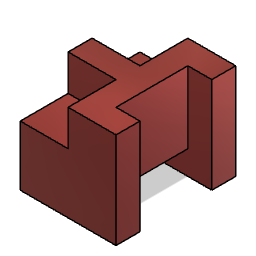
3d09 v1 (Autodesk Fusion 360 design; units mm, degrees)
Autodesk Fusion 360 part; units mm, degrees
sketch "Sketch1" plane through (0, 0, 0) normal (0, 0, 1) x (1, 0, 0)
  line L0 (0, 0) -> (0, 25)
  line L1 (0, 25) -> (20, 25)
  line L2 (20, 25) -> (20, 40)
  line L3 (20, 40) -> (40, 40)
  line L4 (40, 40) -> (40, 0)
  line L5 (40, 0) -> (0, 0)
  dimension "d1" = 40
  dimension "d2" = 25
  dimension "d3" = 20
  dimension "d4" = 15
  constraint coincident L0.start L5.end
  constraint vertical L0
  constraint perpendicular L0 L1
  constraint perpendicular L1 L2
  constraint perpendicular L2 L3
  constraint perpendicular L3 L4
  constraint perpendicular L0 L5
  measures "d1" distance of L4.end L0.start
  measures "d2" distance of L0.start L0.end
  measures "d3" distance of L2.end L3.end
  measures "d4" distance of L1.end L2.end
extrude "Extrude1" add sketch "Sketch1" along normal mid plane 50
sketch "Sketch2" plane through (0, 0, 0) normal (0, 0, 1) x (1, 0, 0)
  line L0 (0, 40) -> (20, 40)
  line L1 (20, 40) -> (20, 25)
  line L2 (20, 25) -> (0, 25)
  line L3 (0, 25) -> (0, 40)
  point P0 (20, 25)
  point P1 (0, 25)
  dimension "d7" = 20
  dimension "d8" = 15
  constraint horizontal L0
  constraint vertical L1
  constraint horizontal L2
  constraint vertical L3
  constraint coincident L1 P0
  constraint coincident L2 P1
  measures "d7" distance of L0.start L0.end
  measures "d8" distance of L0.start L2.end
extrude "Extrude2" add sketch "Sketch2" along normal mid plane 10
sketch "Sketch3" plane through (0, 40, 0) normal (0, 1, 0) x (-1, 0, 0)
  line L0 (-20, -25) -> (-20, -5)
  line L1 (-20, -5) -> (0, -5)
  line L2 (0, -5) -> (0, 5)
  line L3 (0, 5) -> (-20, 5)
  line L4 (-20, 5) -> (-20, 25)
  line L5 (-20, 25) -> (-40, 25)
  line L6 (-40, 25) -> (-40, -25)
  line L7 (-40, -25) -> (-20, -25)
  line L8 (-40, -15) -> (-30, -15)
  line L9 (-30, -15) -> (-30, 15)
  line L10 (-30, 15) -> (-40, 15)
  line L11 (-40, 15) -> (-40, -15)
  dimension "d11" = 10
  dimension "d12" = 10
  dimension "d13" = 30
  dimension "d14" = 10
  constraint horizontal L8
  constraint vertical L9
  constraint horizontal L10
  constraint vertical L11
  constraint coincident L6 L8.start
  measures "d11" distance of L8.start L8.end
  measures "d12" distance of L9.end L10.end
  measures "d13" distance of L8.end L9.end
  measures "d14" distance of L5 L10
extrude "Extrude3" cut sketch "Sketch3" against normal blind 85 contours L6 L8 L9 L10 L11
sketch "Sketch4" plane through (0, 0, 0) normal (1, 0, 0) x (0, 0, -1)
  line L0 (15, 0) -> (15, 10)
  line L1 (15, 10) -> (-15, 10)
  line L2 (-15, 10) -> (-15, 0)
  line L3 (25, 0) -> (-25, 0)
  dimension "d17" = 10
  dimension "d18" = 10
  dimension "d19" = 10
  dimension "d20" = 30
  constraint vertical L0
  constraint perpendicular L0 L1
  constraint perpendicular L1 L2
  constraint coincident L2.end L3
  measures "d17" distance of L1.end L2.end
  measures "d18" distance of L0.start L0.end
  measures "d19" distance of L0.start L3.start
  measures "d20" distance of L0.end L1.end
extrude "Extrude4" cut sketch "Sketch4" along normal blind 88
